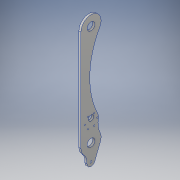
# Autodesk Inventor part: Intake Arm Left
Saved by Autodesk Inventor 2019.4 (Build 234330000, 330)
## iProperties
Created: 2020-01-05
Part Number: Intake Arm Left
Material: Aluminum 6061
Document SubType Name: Modeling
Designer: admin
Density: 2.7 g/cm^3
Appearance: Aluminum - Flat
Author: admin
Autodesk Inventor part; units mm, degrees
ref_plane "YZ Plane" through (0, 0, 0) normal (1, 0, 0) x (0, 1, 0)
ref_plane "XZ Plane" through (0, 0, 0) normal (0, 1, 0) x (-1, 0, 0)
ref_plane "XY Plane" through (0, 0, 0) normal (0, 0, 1) x (1, 0, 0)
sketch "Sketch1" plane through (0, 0, 0) normal (1, 0, 0) x (0, 1, 0)
  line L0 (0, 0) -> (41.1438, 0) construction
  line L1 (41.1438, -41.1438) -> (0, 0) construction
  line L2 (41.1438, -91.1438) -> (0, 0) construction
  line L3 (41.1438, 0) -> (41.1438, -41.1438) construction
  line L4 (41.1438, -91.1438) -> (41.1438, -41.1438) construction
  circle A0 centre (41.1438, 0) radius 9.55
  circle A1 centre (291.1438, 0) radius 9.55
  circle A2 centre (0, 0) radius 2.5
  arc A3 (279.0328, -21.8706) -> (291.1438, 25) centre (291.1438, 0) ccw
  arc A4 (41.1438, 25) -> (23.9214, 18.1215) centre (41.1438, 0) ccw
  arc A5 (-3.6458, -9.3117) -> (0.8136, 9.9668) centre (0, 0) ccw construction
  arc A6 (0.8136, 9.9668) -> (23.9214, 18.1215) centre (3.2546, 39.8674) ccw
  line L5 (41.1438, 25) -> (291.1438, 25)
  line L6 (-3.6458, -9.3117) -> (32.0294, -23.2793)
  arc A7 (0.8136, 9.9668) -> (-3.6458, -9.3117) centre (0, 0) ccw
  arc A8 (52.2034, -22.4206) -> (41.1438, 25) centre (41.1438, 0) ccw construction
  arc A9 (23.9214, 18.1215) -> (32.0294, -23.2793) centre (41.1438, 0) ccw construction
  arc A10 (32.0294, -23.2793) -> (52.2034, -22.4206) centre (41.1438, 0) ccw
  arc A11 (291.1438, 25) -> (279.0328, -21.8706) centre (291.1438, 0) ccw construction
  circle A12 centre (94.2878, 0) radius 6.5
  arc A13 (95.3192, -16.6657) -> (83.7863, -18.1656) centre (87.2878, 0) ccw construction
  line L7 (87.2878, 0) -> (94.2878, 0) construction
  line L8 (94.2878, 0) -> (291.1438, 0) construction
  arc A14 (279.0328, -21.8706) -> (95.3192, -16.6657) centre (182.1452, -196.8358) ccw
  arc A15 (83.7863, -18.1656) -> (52.2034, -22.4206) centre (74.3227, -67.2619) ccw
  arc A16 (83.7863, -18.1656) -> (95.3192, -16.6657) centre (87.2878, 0) ccw
  line L9 (87.2878, -15.5) -> (73.8644, -7.75) construction
  line L10 (73.8644, -7.75) -> (73.8644, 7.75) construction
  line L11 (73.8644, 7.75) -> (87.2878, 15.5) construction
  line L12 (87.2878, 15.5) -> (100.7112, 7.75) construction
  line L13 (100.7112, 7.75) -> (100.7112, -7.75) construction
  line L14 (100.7112, -7.75) -> (87.2878, -15.5) construction
  circle A17 centre (87.2878, -15.5) radius 1.5
  circle A18 centre (73.8644, -7.75) radius 1.5
  circle A19 centre (73.8644, 7.75) radius 1.5
  circle A20 centre (87.2878, 15.5) radius 1.5
  circle A21 centre (100.7112, 7.75) radius 1.5
  circle A22 centre (100.7112, -7.75) radius 1.5
  dimension "d1" = 50
  dimension "d2" = 100
  dimension "d3" = 19.1
  dimension "d4" = 19.1
  dimension "d5" = 5
  dimension "d6" = 250
  dimension "d7" = 50
  dimension "d8" = 50
  dimension "d9" = 20
  dimension "d10" = 30
  dimension "d14" = 13
  dimension "d15" = 7
  dimension "d16" = 37
  dimension "d17" = 200
  dimension "d18" = 50
  dimension "d19" = 31
  dimension "d20" = 3
  dimension "d21" = 3
  dimension "d22" = 3
  dimension "d23" = 3
  dimension "d24" = 3
  dimension "d25" = 3
  dimension "d26" = 203.856
  constraints: 30 end point, 27 point on circle, 23 centre point, 13 tangent, 12 coincident, 3 horizontal, 2 vertical, 1 collinear, 1 perpendicular, 1 point on line, 13 other
  measures "d1" distance of L2.start L1.start
  measures "d2" distance of L2.start L0.start
  measures "d3" diameter of A0
  measures "d4" diameter of A1
  measures "d5" diameter of A2
  measures "d6" distance of A1.centre A0.centre
  measures "d7" diameter of A3
  measures "d8" diameter of A4
  measures "d9" diameter of A5
  measures "d10" radius of A6
  measures "d14" diameter of A12
  measures "d15" distance of L7.start L7.end
  measures "d16" diameter of A13
  measures "d17" radius of A14
  measures "d18" radius of A15
  measures "d19" distance of L9.start L11.end
  measures "d20" diameter of A17
  measures "d21" diameter of A18
  measures "d22" diameter of A19
  measures "d23" diameter of A20
  measures "d24" diameter of A21
  measures "d25" diameter of A22
  measures "d26" distance of L8.end L7.start
extrude "Extrusion1" add sketch "Sketch1" along normal blind 5
body "Solid1"
